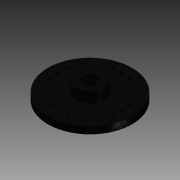
# Autodesk Inventor part: Servo wheel
Saved by Autodesk Inventor 2015 (Build 190159000, 159)
## iProperties
Created: 2015-02-28
Part Number: Servo wheel
Material: Generic
Document SubType Name: Modeling
Designer: Henke
Density: 1 g/cm^3
Appearance: Fine Textured - Black
Mass: 0.534071 g
Surface Area: 7.71261 cm^2
Volume: 0.534071 cm^3
Author: Henke
Autodesk Inventor part; units mm, degrees
ref_plane "YZ Plane" through (0, 0, 0) normal (1, 0, 0) x (0, 1, 0)
ref_plane "XZ Plane" through (0, 0, 0) normal (0, 1, 0) x (-1, 0, 0)
ref_plane "XY Plane" through (0, 0, 0) normal (0, 0, 1) x (1, 0, 0)
sketch "Sketch1" plane through (0, 0, 0) normal (0, 1, 0) x (-1, 0, 0)
  circle A0 centre (0, 0) radius 12
  dimension "d0" = 24
  constraints: 1 centre point, 1 coincident
  measures "d0" diameter of A0
extrude "Extrusion1" add sketch "Sketch1" along normal blind 2
sketch "Sketch2" plane through (0, 2, 0) normal (0, 1, 0) x (1, 0, 0)
  circle A0 centre (0, 0) radius 4
  dimension "d3" = 8
  constraints: 1 centre point, 1 coincident
  measures "d3" diameter of A0
extrude "Extrusion2" add sketch "Sketch2" along normal blind 3
sketch "Sketch3" plane through (0, 5, 0) normal (0, 1, 0) x (1, 0, 0)
  point P0 (0, 0)
  point P1 (0, 0)
  constraints: 1 coincident
hole "Hole1" at (0, 5, 0) direction (0, -1, 0) diameter 3 end through all counterbore diameter 4 counterbore depth 1
sketch "Sketch4" plane through (0, 2, 0) normal (0, 1, 0) x (1, 0, 0)
  circle A0 centre (-9.25, 0) radius 0.5
  line L0 (0, 0) -> (-9.25, 0) construction
  line L1 (0, 0) -> (-9.1094, 2.4408) construction
  line L2 (0, 0) -> (-9.1094, -2.4408) construction
  circle A1 centre (-9.1094, 2.4408) radius 0.5
  circle A2 centre (-9.1094, -2.4408) radius 0.5
  circle A3 centre (0, 0) radius 12 projected
  circle A4 centre (12, 0) radius 21.25 construction
  dimension "d13" = 15
  dimension "d14" = 15
  dimension "d15" = 1
  dimension "d16" = 1
  dimension "d17" = 1
  dimension "d25" = 9.25
  constraints: 6 end point, 4 centre point, 3 point on circle, 2 coincident, 1 horizontal, 1 horizontal alignment, 1 point on line, 1 other
  measures "d13" angle of L0 L2
  measures "d14" angle of L0 L1
  measures "d15" diameter of A1
  measures "d16" diameter of A2
  measures "d17" diameter of A0
  measures "d25" distance of L0.start L0.end
extrude "Extrusion3" cut sketch "Sketch4" against normal through all contours A0 | A1 | A2
pattern_circular "Circular Pattern1" count 4 over 360 about axis through (0, -29.8074, 0) along (0, 1, 0) of "Extrusion3"
body "Solid1"
